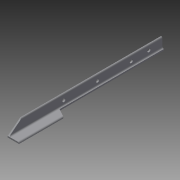
# Autodesk Inventor part: 2x2 quarter in angle aluminum number 2
Saved by Autodesk Inventor 2015 (Build 190159000, 159)
## iProperties
Created: 2015-02-01
Part Number: 2x2 quarter in angle aluminum number 2
Material: Generic
Document SubType Name: Modeling
Designer: szymsea16
Density: 1 g/cm^3
Appearance: Default
Author: szymsea16
Autodesk Inventor part; units mm, degrees
ref_plane "YZ Plane" through (0, 0, 0) normal (1, 0, 0) x (0, 1, 0)
ref_plane "XZ Plane" through (0, 0, 0) normal (0, 1, 0) x (-1, 0, 0)
ref_plane "XY Plane" through (0, 0, 0) normal (0, 0, 1) x (1, 0, 0)
sketch "Sketch1" plane through (0, 0, 0) normal (0, 1, 0) x (-1, 0, 0)
  line L0 (0, 0) -> (50.8, 0)
  line L1 (50.8, 0) -> (50.8, -736.6)
  line L2 (50.8, -736.6) -> (0, -736.6)
  line L3 (0, -736.6) -> (0, 0)
  dimension "d0" = 50.8
  dimension "d1" = 736.6
  constraints: 8 end point, 2 horizontal, 1 parallel, 1 perpendicular
  measures "d0" distance of L0.start L0.end
  measures "d1" distance of L0.end L1.end
extrude "Extrusion1" add sketch "Sketch1" along normal blind 6.35
sketch "Sketch2" plane through (0, 6.35, 0) normal (0, 1, 0) x (1, 0, 0)
  line L0 (-50.8, 0) -> (-44.45, 0)
  line L1 (-50.8, 0) -> (0, 0) projected
  line L2 (-44.45, 0) -> (-44.45, 736.6)
  line L3 (0, 736.6) -> (-50.8, 736.6) projected
  line L4 (-44.45, 736.6) -> (-50.8, 736.6)
  line L5 (-50.8, 736.6) -> (-50.8, 0)
  line L6 (-50.8, 0) -> (-44.45, 0)
  dimension "d4" = 6.35
  dimension "d5" = 736.6
  dimension "d6" = 736.6
  constraints: 10 end point, 1 perpendicular, 1 point on line, 1 vertical
  measures "d4" distance of L0.start L0.end
  measures "d5" distance of L0.end L2.end
  measures "d6" distance of L3.end L0.start
extrude "Extrusion2" add sketch "Sketch2" along normal blind 44.45
fillet "Fillet1" radius 6.35 1 edges at (-44.45, 6.35, -368.3)
fillet "Fillet2" radius 6.35 1 edges at (0, 6.35, -368.3)
fillet "Fillet3" radius 6.35 1 edges at (-44.45, 50.8, -368.3)
hole "Hole1" at (-44.45, 25.4, -247.65) direction (-1, 0, 0) diameter 14.605 end through all
pattern_linear "Rectangular Pattern1" count 3 spacing 152.4 along (0, 0, -1) of "Hole1"
hole "Hole2" at (-44.45, 28.575, -632.1298) direction (-1, 0, 0) diameter 15.24 end through all
sketch "Sketch4" plane through (0, 6.35, 0) normal (0, 1, 0) x (1, 0, 0)
  line L0 (-6.35, 736.6) -> (-6.35, 0) projected
  line L1 (-6.35, 736.6) -> (-38.1, 736.6) projected
  line L2 (-38.1, 0) -> (-38.1, 736.6) projected
  line L3 (-38.1, 0) -> (-6.35, 0) projected
  line L4 (0, 736.6) -> (0, 0) projected
  line L5 (-50.8, 736.6) -> (-50.8, 0) projected
  line L6 (-38.1, 0) -> (-38.1, 736.6) projected
  line L7 (-38.1, 703.0986) -> (0, 703.0986)
  line L8 (0, 703.0986) -> (0, 221.796)
  line L9 (0, 221.796) -> (-38.1, 221.796)
  line L10 (-38.1, 221.796) -> (-38.1, 703.0986)
  line L11 (-38.1, 221.796) -> (0, 200.8397)
  line L12 (0, 221.796) -> (-38.1, 221.796)
  line L13 (0, 221.796) -> (0, 200.8397)
  constraints: 14 end point, 3 point on line, 2 collinear, 2 parallel, 1 horizontal, 1 perpendicular
extrude "Extrusion3" cut sketch "Sketch4" against normal blind 25.4 contours L7 L4 L9 L0 | L0 L9 L2 L7 | L9 L4 L11 L0 | L0 L11 L9
sketch "Sketch7" plane through (-50.8, 0, -736.6) normal (-1, 0, 0) x (0, 0, 1)
  line L0 (736.6, 0) -> (736.6, 50.8) projected
  line L1 (736.6, 19.05) -> (658.9663, 96.6837)
  line L2 (736.6, 19.05) -> (846.3906, 19.05) construction
  line L3 (658.9663, 96.6837) -> (839.9542, 96.6837)
  line L4 (839.9542, 96.6837) -> (736.6, 19.05)
  dimension "d37" = 135
  constraints: 8 end point, 1 equal length, 1 horizontal, 1 perpendicular, 1 point on line
  measures "d37" angle of L2 L1
extrude "Extrusion4" cut sketch "Sketch7" against normal blind 25.4
sketch "Sketch8" plane through (-44.45, 12.7, 0) normal (1, 0, 0) x (0, 0, -1)
  line L0 (693.0898, 15.875) -> (693.0898, 61.5765)
  line L1 (693.0898, 61.5765) -> (693.0898, -44.6124)
  line L2 (693.0898, -44.6124) -> (800.4585, -39.8743)
  line L3 (800.4585, -39.8743) -> (791.1289, 38.6781)
  line L4 (791.1289, 38.6781) -> (744.7163, 67.7082)
  line L5 (744.7163, 67.7082) -> (693.0898, 61.5765)
  point P0 (0, -12.7)
  constraints: 12 end point, 1 perpendicular, 1 point on line
extrude "Extrusion5" cut sketch "Sketch8" along normal mid plane 96.8375
sketch "Sketch9" plane through (-50.8, 0, 0) normal (-1, 0, 0) x (0, 0, 1)
  line L0 (0, 0) -> (0, 6.35)
  line L1 (0, 6.35) -> (-221.796, 6.35) projected
  line L2 (-31.75, 50.8) -> (-57.15, 50.8)
  line L3 (-693.0898, 50.8) -> (-31.75, 50.8) projected
  line L4 (-57.15, 50.8) -> (0, 6.35)
  line L5 (37.7088, 23.9935) -> (15.7268, 85.5344)
  line L6 (15.7268, 85.5344) -> (-31.75, 88.3696)
  line L7 (-31.75, 88.3696) -> (-57.15, 50.8)
  line L8 (37.7088, 23.9935) -> (0, 6.35)
  dimension "d43" = 6.35
  dimension "d44" = 25.4
  constraints: 14 end point, 1 perpendicular, 1 point on line
  measures "d43" distance of L0.start L0.end
  measures "d44" distance of L2.start L2.end
extrude "Extrusion6" cut sketch "Sketch9" against normal blind 96.8375
body "Solid1"
